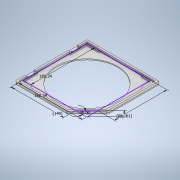
# Autodesk Inventor part: Box_Walls_2
Saved by Autodesk Inventor 2022 (Build 260153000, 153)
## iProperties
Created: 2023-02-27
Part Number: Box_Walls_2
Material: Generic
Document SubType Name: Modeling
Designer: zarek
Density: 1 g/cm^3
Appearance: Default
Author: zarek
Autodesk Inventor part; units mm, degrees
ref_plane "YZ Plane" through (0, 0, 0) normal (1, 0, 0) x (0, 1, 0)
ref_plane "XZ Plane" through (0, 0, 0) normal (0, 1, 0) x (-1, 0, 0)
ref_plane "XY Plane" through (0, 0, 0) normal (0, 0, 1) x (1, 0, 0)
sketch "Sketch1" plane through (0, 0, 0) normal (0, 1, 0) x (-1, 0, 0)
  line L0 (101.6, -101.6) -> (-101.6, -101.6)
  line L1 (-101.6, -101.6) -> (-101.6, 101.6)
  line L2 (-101.6, 101.6) -> (101.6, 101.6)
  line L3 (101.6, 101.6) -> (101.6, -101.6)
  line L4 (96.6, -96.6) -> (-96.6, -96.6)
  line L5 (-96.6, -96.6) -> (-96.6, 96.6)
  line L6 (-96.6, 96.6) -> (96.6, 96.6)
  line L7 (96.6, 96.6) -> (96.6, -96.6)
  line L8 (101.6, 101.6) -> (-40.4, 101.6)
  circle A0 centre (0, 0) radius 86.4
  circle A1 centre (0, 0) radius 109.3376
  line L9 (-40.4, 101.6) -> (-101.6, 40.4)
  line L10 (-45.4, 101.6) -> (-101.6, 45.4)
  line L11 (96.6, 96.6) -> (96.6, 101.6)
  line L12 (-45.4, 101.6) -> (-35.4, 101.6)
  line L13 (-35.4, 101.6) -> (-35.4, 96.6)
  line L14 (-35.4, 96.6) -> (-45.4, 96.6)
  line L15 (-45.4, 96.6) -> (-45.4, 101.6)
  circle A2 centre (0, 0) radius 111.3376
  point P0 (96.6, 51.2168)
  point P1 (101.6, 40.4)
  point P2 (101.6, -40.4)
  point P3 (96.6, -51.2168)
  point P4 (-96.6, 45.4)
  point P5 (-45.4, 96.6)
  dimension "d0" = 203.2
  dimension "d1" = 203.2
  dimension "d2" = 101.6
  dimension "d3" = 101.6
  dimension "d4" = 5
  dimension "d5" = 5
  dimension "d6" = 5
  dimension "d7" = 5
  dimension "d10" = 142
  dimension "d12" = 61.2
  dimension "d14" = 172.8
  dimension "d15" = 5
  dimension "d16" = 5
  dimension "d17" = 10
  dimension "d34" = 2
  constraints: 32 end point, 7 parallel, 6 point on line, 4 perpendicular, 3 centre point, 3 coincident, 3 horizontal, 2 point on circle
  measures "d0" distance between parallel lines of L2 L0
  measures "d1" distance between parallel lines of L1 L3
  measures "d2" distance from line of L0 point (0, 0)
  measures "d3" distance from line of L1 point (0, 0)
  measures "d4" distance between parallel lines of L4 L0
  measures "d5" distance between parallel lines of L1 L5
  measures "d6" distance between parallel lines of L2 L6
  measures "d7" distance between parallel lines of L3 L7
  measures "d10" distance of L2.end L8.end
  measures "d12" distance from line of L1 L8.end
  measures "d14" diameter of A0
  measures "d15" distance of L10.end L9.end
  measures "d16" distance of L10.start L8.end
  measures "d17" distance of L13.end L14.end
  measures "d34" radial gap between concentric circles of A1 A2
extrude "Extrusion1" add sketch "Sketch1" along normal blind 3 contours L0 A2 L4 L7 L3 | L0 A1 L4 A2 | A2 L7 A1 L3 | L0 A1 L4 | A2 L4 A1 L0 | L0 L1 A2 L5 L4 | A2 L7 L4 | L4 A1 L7 A2 | A1 L7 L3 | L4 A1 L5 L9 L6 L7 | A2 L5 A1 L4 | L4 L5 A2 | A1 L7 A2 L3 | A2 L7 L11 L2 L3 | L1 A1 L5 A2 | A1 L6 A2 L7 | A2 L6 L7 | A1 L1 L9 L5 | A1 L2 A2 L6 | L6 L13 L2 A1 | L11 L6 A2 L2 | L9 A1 L10 L5 | L5 L10 L6 L9 | L1 L10 A1 | L6 L9 L2 L13 | L15 A1 L9 | L6 L10 A1 L15 | A1 L15 L2 | A1 L10 L15
sketch "Sketch5" plane through (0, 3, 0) normal (0, 1, 0) x (1, 0, 0)
  line L0 (-101.6, 101.6) -> (101.6, 101.6)
  line L1 (101.6, 101.6) -> (101.6, -101.6)
  line L2 (101.6, -101.6) -> (-101.6, -101.6)
  line L3 (-101.6, -101.6) -> (-101.6, 101.6)
  line L4 (-96.6, 96.6) -> (96.6, 96.6)
  line L5 (96.6, 96.6) -> (96.6, -96.6)
  line L6 (96.6, -96.6) -> (-96.6, -96.6)
  line L7 (-96.6, -96.6) -> (-96.6, 96.6)
  line L8 (-101.6, -101.6) -> (40.4, -101.6)
  circle A0 centre (0, 0) radius 88.9
  circle A1 centre (0, 0) radius 109.3376
  line L9 (40.4, -101.6) -> (101.6, -40.4)
  line L10 (45.4, -101.6) -> (101.6, -45.4)
  line L11 (-96.6, -96.6) -> (-96.6, -101.6)
  line L12 (45.4, -101.6) -> (35.4, -101.6)
  line L13 (35.4, -101.6) -> (35.4, -96.6)
  line L14 (35.4, -96.6) -> (45.4, -96.6)
  line L15 (45.4, -96.6) -> (45.4, -101.6)
  circle A2 centre (0, 0) radius 111.3376
  point P0 (96.6, 101.6)
  point P1 (96.6, 51.2168)
  point P2 (101.6, 40.4)
  point P3 (101.6, -40.4)
  point P4 (96.6, -51.2168)
  point P5 (-96.6, 45.4)
  point P6 (-45.4, 96.6)
  point P7 (-35.4, 101.6)
  point P8 (-55.358, -96.6)
  point P9 (-96.6, -55.358)
  point P10 (-96.6, 55.358)
  point P11 (-55.358, 96.6)
  point P12 (55.358, 96.6)
  point P13 (96.6, 55.358)
  point P14 (96.6, -45.4)
  point P15 (45.4, -96.6)
  dimension "d37" = 203.2
  dimension "d38" = 203.2
  dimension "d39" = 101.6
  dimension "d40" = 101.6
  dimension "d41" = 5
  dimension "d42" = 5
  dimension "d43" = 5
  dimension "d44" = 5
  dimension "d45" = 142
  dimension "d46" = 61.2
  dimension "d47" = 177.8
  dimension "d48" = 5
  dimension "d49" = 5
  dimension "d50" = 10
  dimension "d51" = 2
  constraints: 32 end point, 7 parallel, 6 point on line, 4 perpendicular, 3 centre point, 3 coincident, 2 point on circle
  measures "d37" distance between parallel lines of L2 L0
  measures "d38" distance between parallel lines of L1 L3
  measures "d39" distance from line of L0 point (0, 0)
  measures "d40" distance from line of L1 point (0, 0)
  measures "d41" distance between parallel lines of L4 L0
  measures "d42" distance between parallel lines of L1 L5
  measures "d43" distance between parallel lines of L2 L6
  measures "d44" distance between parallel lines of L3 L7
  measures "d45" distance of L2.end L8.end
  measures "d46" distance from line of L1 L8.end
  measures "d47" diameter of A0
  measures "d48" distance of L10.end L9.end
  measures "d49" distance of L10.start L8.end
  measures "d50" distance of L13.end L14.end
  measures "d51" radial gap between concentric circles of A1 A2
extrude "Extrusion4" add sketch "Sketch5" along normal blind 3 contours L0 A2 L4 L7 L3 | L0 A1 L4 A2 | A2 L7 A1 L3 | L0 A1 L4 | A2 L4 A1 L0 | L0 L1 A2 L5 L4 | A2 L7 L4 | A1 L7 L3 | A2 L7 L11 L2 L3 | L3 A1 L7 A2 | L4 L5 A2 | A2 L6 L7 | L1 A1 L5 A2 | L11 L6 A2 L2 | L6 A1 L2 A2 | A1 L1 L9 L5 | L6 L13 L2 A1 | L9 A1 L10 L5 | L5 L10 L6 L9 | L1 L10 A1 | L6 L9 L2 L13 | L15 A1 L9 | L6 L10 A1 L15 | A1 L15 L2 | L15 A1 L10
sketch "Sketch6" plane through (0, 6, 0) normal (0, 1, 0) x (1, 0, 0)
  line L0 (-101.6, 101.6) -> (101.6, 101.6)
  line L1 (101.6, 101.6) -> (101.6, -101.6)
  line L2 (101.6, -101.6) -> (-101.6, -101.6)
  line L3 (-101.6, -101.6) -> (-101.6, 101.6)
  line L4 (-96.6, 96.6) -> (96.6, 96.6)
  line L5 (96.6, 96.6) -> (96.6, -96.6)
  line L6 (96.6, -96.6) -> (-96.6, -96.6)
  line L7 (-96.6, -96.6) -> (-96.6, 96.6)
  line L8 (-101.6, -101.6) -> (40.4, -101.6)
  circle A0 centre (0, 0) radius 88.9
  circle A1 centre (0, 0) radius 109.3376
  line L9 (40.4, -101.6) -> (101.6, -40.4)
  line L10 (45.4, -101.6) -> (101.6, -45.4)
  line L11 (-96.6, -96.6) -> (-96.6, -101.6)
  line L12 (45.4, -101.6) -> (35.4, -101.6)
  line L13 (35.4, -101.6) -> (35.4, -96.6)
  line L14 (35.4, -96.6) -> (45.4, -96.6)
  line L15 (45.4, -96.6) -> (45.4, -101.6)
  circle A2 centre (0, 0) radius 111.3376
  point P0 (96.6, 101.6)
  point P1 (96.6, 51.2168)
  point P2 (101.6, 40.4)
  point P3 (101.6, -40.4)
  point P4 (96.6, -51.2168)
  point P5 (-96.6, 45.4)
  point P6 (-45.4, 96.6)
  point P7 (-35.4, 101.6)
  point P8 (55.358, 96.6)
  point P9 (96.6, 55.358)
  point P10 (96.6, -45.4)
  point P11 (45.4, -96.6)
  dimension "d54" = 203.2
  dimension "d55" = 203.2
  dimension "d56" = 101.6
  dimension "d57" = 101.6
  dimension "d58" = 5
  dimension "d59" = 5
  dimension "d60" = 5
  dimension "d61" = 5
  dimension "d62" = 142
  dimension "d63" = 61.2
  dimension "d64" = 177.8
  dimension "d65" = 5
  dimension "d66" = 5
  dimension "d67" = 10
  dimension "d68" = 2
  constraints: 32 end point, 7 parallel, 6 point on line, 4 perpendicular, 3 centre point, 3 coincident, 2 point on circle
  measures "d54" distance between parallel lines of L2 L0
  measures "d55" distance between parallel lines of L1 L3
  measures "d56" distance from line of L0 point (0, 0)
  measures "d57" distance from line of L1 point (0, 0)
  measures "d58" distance between parallel lines of L4 L0
  measures "d59" distance between parallel lines of L1 L5
  measures "d60" distance between parallel lines of L2 L6
  measures "d61" distance between parallel lines of L3 L7
  measures "d62" distance of L2.end L8.end
  measures "d63" distance from line of L1 L8.end
  measures "d64" diameter of A0
  measures "d65" distance of L10.end L9.end
  measures "d66" distance of L10.start L8.end
  measures "d67" distance of L13.end L14.end
  measures "d68" radial gap between concentric circles of A1 A2
extrude "Extrusion5" add sketch "Sketch6" along normal blind 3.5 contours L0 A2 L4 L7 L3 | L0 A1 L4 A2 | A2 L7 A1 L3 | L0 A1 L4 | A2 L4 A1 L0 | L0 L1 A2 L5 L4 | A1 L7 L3 | A2 L7 L11 L2 L3 | L3 A1 L7 A2 | L1 A1 L5 A2 | L11 L6 A2 L2 | L6 A1 L2 A2 | A1 L1 L9 L5 | L6 L13 L2 A1 | L9 A1 L10 L5 | L5 L10 L6 L9 | L1 L10 A1 | L6 L9 L2 L13 | L15 A1 L9 | L6 L10 A1 L15 | A1 L15 L2 | L15 A1 L10
fillet "Fillet6" radius 3.175 5 edges at (-28.1, 0, 101.6) (73.5, 0, 73.5) (101.6, 0, -28.1) (0, 0, -101.6) (-101.6, 0, 0)
sketch "Sketch7" plane through (0, 0, 0) normal (0, -1, 0) x (1, 0, 0)
  line L0 (101.6, 45.4) -> (101.6, -101.6) projected
  line L1 (98.425, 44.0849) -> (98.425, -98.425) projected
  line L2 (101.6, -101.6) -> (98.425, -101.6)
  line L3 (98.425, -101.6) -> (98.425, 39.0849)
  line L4 (98.425, 39.0849) -> (101.6, 39.0849)
  line L5 (101.6, 39.0849) -> (101.6, -101.6)
  line L6 (44.0849, 98.425) -> (98.425, 44.0849) projected
  line L7 (98.425, 44.0849) -> (101.6, 44.0849)
  point P0 (0, 0)
  dimension "d73" = 5
  constraints: 10 end point, 2 horizontal, 2 parallel, 2 point on line, 1 perpendicular
  measures "d73" distance between parallel lines of L4 L7
extrude "Extrusion6" add sketch "Sketch7" against normal blind 3 contours L0 L2 L3 L1 L4
fillet "Fillet7" radius 3.175 1 edges at (100.0125, 0, -101.6)
fillet "Fillet8" radius 3.175 4 edges at (-100.6701, 0.9299, 100.6701) (-101.6, 6.3375, 101.6) (-100.6701, 0.9299, -100.6701) (-101.6, 6.3375, -101.6)
fillet "Fillet9" radius 3.175 4 edges at (100.6701, 0.9299, 45.0148) (101.6, 6.3375, 45.4) (45.0148, 0.9299, 100.6701) (45.4, 6.3375, 101.6)
sketch "Sketch11" plane through (0, 3, 0) normal (0, 1, 0) x (1, 0, 0)
  arc A0 (-101.6, -98.425) -> (-98.425, -101.6) centre (-98.425, -98.425) ccw
  line L0 (44.0849, 101.6) -> (-98.425, 101.6)
  line L1 (-101.6, 98.425) -> (-101.6, -98.425)
  line L2 (-101.6, -46.1) -> (-101.6, -76.6)
  line L3 (-96.6, -96.6) -> (-96.6, 96.6)
  line L4 (-96.6, -46.1) -> (-96.6, -76.6)
  line L5 (-101.6, -76.6) -> (-96.6, -76.6)
  line L6 (-101.6, -46.1) -> (-96.6, -46.1)
  line L7 (-98.425, -101.6) -> (101.6, -101.6)
  line L8 (0, 0) -> (-101.6, 0)
  line L9 (-101.6, 46.1) -> (-101.6, 76.6)
  line L10 (-96.6, 46.1) -> (-96.6, 76.6)
  line L11 (-101.6, 76.6) -> (-96.6, 76.6)
  line L12 (-101.6, 46.1) -> (-96.6, 46.1)
  line L13 (-96.6, -76.6) -> (-90.1, -76.6)
  line L14 (-90.1, -76.6) -> (-90.1, -46.1)
  line L15 (-90.1, -46.1) -> (-96.6, -46.1)
  line L16 (-96.6, -46.1) -> (-96.6, -76.6)
  line L17 (-96.6, 46.1) -> (-90.1, 46.1)
  line L18 (-90.1, 46.1) -> (-90.1, 76.6)
  line L19 (-90.1, 76.6) -> (-96.6, 76.6)
  line L20 (-96.6, 76.6) -> (-96.6, 46.1)
  point P0 (-98.425, 98.425)
  point P1 (46.1, 101.6)
  point P2 (46.1, 96.6)
  point P3 (76.6, 96.6)
  point P4 (76.6, 101.6)
  point P5 (-46.1, 96.6)
  point P6 (-96.6, -46.1)
  point P7 (-101.6, 46.1)
  point P8 (-96.6, 46.1)
  point P9 (-96.6, 76.6)
  point P10 (-101.6, 76.6)
  point P11 (-96.6, 76.6)
  dimension "d97" = 30.5
  dimension "d98" = 25
  dimension "d99" = 5
  dimension "d100" = 6.5
  dimension "d101" = 6.5
  constraints: 42 end point, 5 parallel, 5 symmetric about line, 3 perpendicular, 3 point on line, 2 horizontal, 2 point on circle, 1 centre point, 1 midpoint
  measures "d97" distance between parallel lines of L5 L6
  measures "d98" distance between parallel lines of L5 L7
  measures "d99" distance between parallel lines of L4 L2
  measures "d100" distance of L15.end L14.end
  measures "d101" distance of L19.end L18.end
extrude "Extrusion8" add sketch "Sketch11" along normal up to surface (3 mm away) contours L19 L18 L17 L3 | L15 L14 L13 L3
sketch "Sketch8" plane through (0, 9.5, 0) normal (0, 1, 0) x (1, 0, 0)
  arc A0 (-101.6, -98.425) -> (-98.425, -101.6) centre (-98.425, -98.425) ccw
  line L0 (44.0849, 101.6) -> (-98.425, 101.6)
  line L1 (-101.6, 98.425) -> (-101.6, -98.425)
  line L2 (-101.6, -46.1) -> (-101.6, -76.6)
  line L3 (-96.6, -96.6) -> (-96.6, 96.6)
  line L4 (-96.6, -46.1) -> (-96.6, -76.6)
  line L5 (-101.6, -76.6) -> (-96.6, -76.6)
  line L6 (-101.6, -46.1) -> (-96.6, -46.1)
  line L7 (-98.425, -101.6) -> (101.6, -101.6)
  line L8 (0, 0) -> (-101.6, 0)
  line L9 (-101.6, 46.1) -> (-101.6, 76.6)
  line L10 (-96.6, 46.1) -> (-96.6, 76.6)
  line L11 (-101.6, 76.6) -> (-96.6, 76.6)
  line L12 (-101.6, 46.1) -> (-96.6, 46.1)
  line L13 (-96.6, -76.6) -> (-90.1, -76.6)
  line L14 (-90.1, -76.6) -> (-90.1, -46.1)
  line L15 (-90.1, -46.1) -> (-96.6, -46.1)
  line L16 (-96.6, -46.1) -> (-96.6, -76.6)
  line L17 (-96.6, 46.1) -> (-90.1, 46.1)
  line L18 (-90.1, 46.1) -> (-90.1, 76.6)
  line L19 (-90.1, 76.6) -> (-96.6, 76.6)
  line L20 (-96.6, 76.6) -> (-96.6, 46.1)
  line L21 (-96.6, -76.6) -> (-101.6, -76.6)
  line L22 (-101.6, -76.6) -> (-101.6, -74.1)
  line L23 (-101.6, -74.1) -> (-96.6, -74.1)
  line L24 (-96.6, -74.1) -> (-96.6, -76.6)
  line L25 (-96.6, -96.6) -> (-96.6, 96.6) projected
  line L26 (-101.6, -46.1) -> (-96.6, -46.1)
  line L27 (-96.6, -46.1) -> (-96.6, -48.6)
  line L28 (-96.6, -48.6) -> (-101.6, -48.6)
  line L29 (-101.6, -48.6) -> (-101.6, -46.1)
  line L30 (-101.6, 76.6) -> (-96.6, 76.6)
  line L31 (-96.6, 76.6) -> (-96.6, 74.1)
  line L32 (-96.6, 74.1) -> (-101.6, 74.1)
  line L33 (-101.6, 74.1) -> (-101.6, 76.6)
  line L34 (-101.6, 46.1) -> (-96.6, 46.1)
  line L35 (-96.6, 46.1) -> (-96.6, 48.6)
  line L36 (-96.6, 48.6) -> (-101.6, 48.6)
  line L37 (-101.6, 48.6) -> (-101.6, 46.1)
  point P0 (-98.425, 98.425)
  point P1 (46.1, 101.6)
  point P2 (46.1, 96.6)
  point P3 (76.6, 96.6)
  point P4 (76.6, 101.6)
  point P5 (-46.1, 96.6)
  point P6 (-96.6, -46.1)
  point P7 (-101.6, 46.1)
  point P8 (-96.6, 46.1)
  point P9 (-96.6, 76.6)
  point P10 (-101.6, 76.6)
  point P11 (-96.6, 76.6)
  dimension "d77" = 30.5
  dimension "d78" = 25
  dimension "d79" = 5
  dimension "d82" = 6.5
  dimension "d83" = 6.5
  dimension "d169" = 2.5
  dimension "d170" = 2.5
  dimension "d171" = 2.5
  dimension "d172" = 2.5
  constraints: 74 end point, 13 parallel, 7 perpendicular, 6 horizontal, 5 symmetric about line, 4 point on line, 2 point on circle, 1 centre point, 1 midpoint, 4 other
  measures "d77" distance between parallel lines of L5 L6
  measures "d78" distance between parallel lines of L5 L7
  measures "d79" distance between parallel lines of L4 L2
  measures "d82" distance of L15.end L14.end
  measures "d83" distance of L19.end L18.end
  measures "d169" distance between parallel lines of L28 L26
  measures "d170" distance between parallel lines of L5 L23
  measures "d171" distance of L30.end L31.end
  measures "d172" distance of L35.end L34.end
extrude "Extrusion7" cut sketch "Sketch8" against normal blind 2.2 contours L32 L3 L36 L1 | L28 L3 L23 L1
sketch "Sketch15" plane through (0, 3, 0) normal (0, 1, 0) x (1, 0, 0)
  line L0 (0.1655, 2.1158) -> (-93.0045, 2.1158)
  line L1 (-93.0045, 2.1158) -> (-93.0045, 92.4458)
  line L2 (-93.0045, 92.4458) -> (0.1655, 92.4458)
  line L3 (0.1655, 92.4458) -> (0.1655, 2.1158)
  line L4 (0.1655, 2.1158) -> (-93.0045, 2.1158)
  line L5 (-93.0045, 2.1158) -> (-93.0045, -88.0542)
  line L6 (-93.0045, -88.0542) -> (0.1655, -88.0542)
  line L7 (0.1655, -88.0542) -> (0.1655, 2.1158)
  line L8 (0.1655, -88.0542) -> (87.4955, -88.0542)
  line L9 (87.4955, -88.0542) -> (87.4955, -6.1383)
  line L10 (87.4955, -6.1383) -> (0.1655, -6.1383)
  line L11 (0.1655, -6.1383) -> (0.1655, -88.0542)
  line L12 (87.4955, -6.1383) -> (0.1655, -6.1383)
  line L13 (0.1655, -6.1383) -> (0.1655, 92.4458)
  line L14 (0.1655, 92.4458) -> (87.4955, 92.4458)
  line L15 (87.4955, 92.4458) -> (87.4955, -6.1383)
  line L16 (56.4955, -88.0542) -> (87.4955, -57.0542)
  line L17 (56.4955, -88.0542) -> (100.3361, -88.0542) construction
  point P0 (-90.1, -65.4069)
  dimension "d143" = 93.17
  dimension "d144" = 90.17
  dimension "d147" = 180.5
  dimension "d148" = 45
  dimension "d149" = 149.5
  dimension "d150" = 149.5
  dimension "d151" = 93.17
  dimension "d152" = 98.5841
  dimension "d153" = 180.5
  constraints: 36 end point, 8 parallel, 5 horizontal, 4 perpendicular, 2 point on line, 1 equal length
  measures "d143" distance from line of L1 L0.start
  measures "d144" distance of L6.end L0.start
  measures "d147" distance between parallel lines of L15 L1
  measures "d148" angle of L17 L16
  measures "d149" distance of L5.end L16.start
  measures "d150" distance of L16.end L14.end
  measures "d151" distance between parallel lines of L7 L1
  measures "d152" distance between parallel lines of L10 L2
  measures "d153" distance between parallel lines of L6 L2
extrude "Extrusion9" cut sketch "Sketch15" along normal blind 4 contours L7 L6 L5 L0 | L0 L1 L2 L3 | L3 L14 L15 L10 L7 | L10 L9 L16 L8 L7
sketch "Sketch16" plane through (0, 9.5, 0) normal (0, 1, 0) x (1, 0, 0)
  line L0 (-92.6321, 91.7869) -> (87.7079, 91.7869)
  line L1 (87.7079, 91.7869) -> (87.7079, -88.5531)
  line L2 (87.7079, -88.5531) -> (-92.6321, -88.5531)
  line L3 (-92.6321, -88.5531) -> (-92.6321, 91.7869)
  line L4 (56.3679, -88.5531) -> (87.7079, -57.2131)
  line L5 (56.3679, -88.5531) -> (100.6893, -88.5531) construction
  dimension "d154" = 180.34
  dimension "d155" = 180.34
  dimension "d156" = 45
  dimension "d157" = 149
  dimension "d158" = 149
  dimension "d159" = 22.1607
  constraints: 12 end point, 2 horizontal, 2 parallel, 2 point on line, 1 equal length, 1 perpendicular
  measures "d154" distance between parallel lines of L2 L0
  measures "d155" distance between parallel lines of L1 L3
  measures "d156" angle of L5 L4
  measures "d157" distance of L4.end L0.end
  measures "d158" distance of L4.start L2.end
  measures "d159" distance from line of L4 L1.end
sketch "Sketch17" plane through (0, 3, 0) normal (0, 1, 0) x (1, 0, 0)
  line L0 (96.6, -45.4) -> (45.4, -96.6) projected
  line L1 (45.4, -96.6) -> (45.4, -91.6)
  line L2 (56.4955, -88.0542) -> (87.4955, -57.0542) projected
  line L3 (56.4955, -88.0542) -> (52.9497, -91.6)
  line L4 (44.0849, -98.425) -> (98.425, -44.0849) projected
  line L5 (52.9497, -91.6) -> (45.4, -91.6)
  line L6 (87.4955, -57.0542) -> (91.6, -52.9497)
  line L7 (91.6, -52.9497) -> (91.6, -45.4)
  line L8 (91.6, -45.4) -> (96.6, -45.4)
  point P0 (0, 0)
  point P1 (91.6, -50.4)
  point P2 (50.4, -91.6)
  dimension "d160" = 5
  dimension "d161" = 5
  constraints: 12 end point, 2 perpendicular, 1 horizontal, 1 parallel, 1 point on line, 1 vertical
  measures "d160" distance of L0.end L1.end
  measures "d161" distance of L7.end L0.start
extrude "Extrusion10" cut sketch "Sketch17" along normal blind 4 contours L7 L4 L5 L0 | L7 L6 L2 L3 L5 L4
sketch "Sketch19" plane through (0, 6, 0) normal (0, 1, 0) x (1, 0, 0)
  line L0 (-93.0045, 46.1) -> (-96.6, 46.1) projected
  line L1 (-96.6, 46.1) -> (-94.1, 46.1)
  line L2 (-94.1, 46.1) -> (-94.1, 76.6805)
  line L3 (-94.1, 76.6805) -> (-96.6, 76.6805)
  line L4 (-96.6, 76.6805) -> (-96.6, 46.1)
  line L5 (-101.6, -46.1) -> (-96.6, -46.1) projected
  line L6 (-96.6, -46.1) -> (-94.1, -46.1)
  line L7 (-94.1, -46.1) -> (-94.1, -76.6)
  line L8 (-94.1, -76.6) -> (-96.6, -76.6)
  line L9 (-96.6, -76.6) -> (-96.6, -46.1)
  point P0 (0, 0)
  dimension "d99" = 5
  dimension "d165" = 2.5
  dimension "d168" = 2.5
  constraints: 16 end point, 4 parallel, 2 horizontal, 2 perpendicular
  measures "d165" distance of L3.end L2.end
  measures "d168" distance between parallel lines of L9 L7
extrude "Extrusion11" add sketch "Sketch19" along normal up to surface (1.3 mm away)
sketch "Sketch12" plane through (0, 6, 0) normal (0, 1, 0) x (1, 0, 0)
  line L0 (-94, 94) -> (94, 94)
  line L1 (94, 94) -> (94, -94)
  line L2 (94, -94) -> (-94, -94)
  line L3 (-94, -94) -> (-94, 94)
  circle A0 centre (-94, 94) radius 1
  circle A1 centre (94, 94) radius 1
  circle A2 centre (-94, -94) radius 1
  circle A3 centre (94, -39.0849) radius 1.5
  point P0 (0, 0)
  dimension "d104" = 94
  dimension "d105" = 94
  dimension "d106" = 94
  dimension "d107" = 94
  dimension "d108" = 2
  dimension "d109" = 2
  dimension "d110" = 2
  dimension "d164" = 3
  constraints: 8 end point, 4 centre point, 3 coincident, 2 parallel, 1 horizontal, 1 perpendicular, 1 point on line
  measures "d104" distance from line of point (0, 0) L0
  measures "d105" distance from line of point (0, 0) L3
  measures "d106" distance from line of point (0, 0) L1
  measures "d107" distance from line of L2 point (0, 0)
  measures "d108" diameter of A0
  measures "d109" diameter of A1
  measures "d110" diameter of A2
  measures "d164" diameter of A3
hole "Assembly Holes" at (-94, 6, 94) at (-94, 6, -94) at (94, 6, -94) at (94, 6, 39.0849) direction (0, -1, 0) diameter 2.85 depth 4 tip angle 118 countersink diameter 2.9 countersink angle 90 thread size "M3.5x0.6" class "6H" standard "ANSI Metric M Profile"
sketch "Sketch10" plane through (0, 7.3, 0) normal (0, 1, 0) x (1, 0, 0)
  line L0 (-90.1, -76.6) -> (-90.1, -46.1)
  line L1 (-101.6, -46.1) -> (-96.6, -46.1)
  line L2 (-90.1, -76.6) -> (-90.1, -46.1)
  line L3 (-90.1, -46.1) -> (-101.6, -46.1)
  line L4 (-101.6, -46.1) -> (-101.6, -76.6)
  line L5 (-101.6, -76.6) -> (-90.1, -76.6)
  line L6 (-96.6, -76.6) -> (-90.1, -76.6)
  line L7 (-91.1, -76.6) -> (-91.1, -46.1)
  line L8 (-91.1, -62.066) -> (-96.35, -62.066)
  line L9 (-96.35, -62.066) -> (-96.35, -71.066)
  line L10 (-96.35, -62.066) -> (-96.35, -53.066)
  circle A0 centre (-96.35, -53.066) radius 1
  circle A1 centre (-96.35, -71.066) radius 1
  line L11 (0, 0) -> (-101.6, 0)
  line L12 (-101.6, 98.425) -> (-101.6, -98.425)
  circle A2 centre (-96.35, 71.066) radius 1
  line L13 (-96.35, 62.066) -> (-96.35, 71.066)
  line L14 (-91.1, 62.066) -> (-96.35, 62.066)
  line L15 (-101.6, 76.6) -> (-90.1, 76.6)
  line L16 (-96.35, 62.066) -> (-96.35, 53.066)
  circle A3 centre (-96.35, 53.066) radius 1
  line L17 (-101.6, 46.1) -> (-96.6, 46.1)
  line L18 (-90.1, 46.1) -> (-101.6, 46.1)
  line L19 (-91.1, 76.6) -> (-91.1, 46.1)
  line L20 (-101.6, 46.1) -> (-101.6, 76.6)
  line L21 (-90.1, 76.6) -> (-90.1, 46.1)
  line L22 (-90.1, 76.6) -> (-90.1, 46.1)
  line L23 (-96.6, 76.6) -> (-90.1, 76.6)
  dimension "d84" = 1
  dimension "d85" = 5.25
  dimension "d86" = 9
  dimension "d87" = 9
  dimension "d88" = 2
  dimension "d89" = 2
  constraints: 48 end point, 15 symmetric about line, 6 point on line, 4 centre point, 4 coincident, 2 parallel, 2 perpendicular, 1 midpoint, 2 other
  measures "d84" distance between parallel lines of L0 L7
  measures "d85" distance of L8.start L8.end
  measures "d86" distance of L8.end L9.end
  measures "d87" distance of L8.end L10.end
  measures "d88" diameter of A0
  measures "d89" diameter of A1
hole "Hinge Holes" at (-96.35, 7.3, -71.066) at (-96.35, 7.3, -53.066) at (-96.35, 7.3, 71.066) at (-96.35, 7.3, 53.066) direction (0, -1, 0) diameter 2.85 depth 4 tip angle 118 countersink diameter 2.9 countersink angle 90 thread size "M3.5x0.6" class "6H" standard "ANSI Metric M Profile"
equation "\"d1\" = d0"
equation "\"d2\" = 0.5 * d0"
equation "\"d3\" = 0.5 * d0"
equation "\"d38\" = d37"
equation "\"d39\" = 0.5 * d37"
equation "\"d40\" = 0.5 * d37"
body "Solid1"
